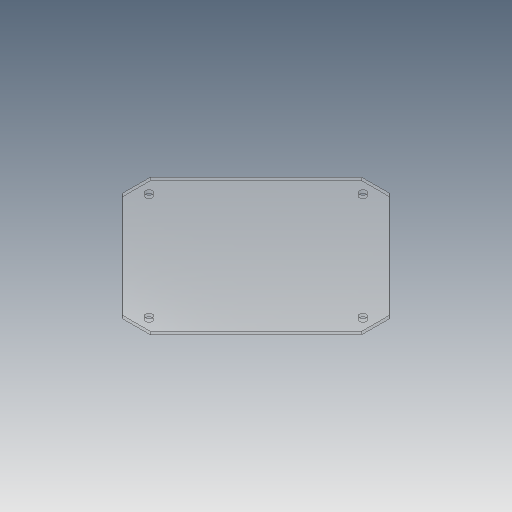
# Autodesk Inventor part: separatingPanels
Saved by Autodesk Inventor 2017 (Build 210142000, 142)
## iProperties
Created: 2016-07-21
Part Number: separatingPanels
Material: Polycarbonate, Clear
Document SubType Name: Modeling
Designer: Jonathan
Density: 1.2 g/cm^3
Appearance: Polycarbonate - Clear
Author: Jonathan
Autodesk Inventor part; units mm, degrees
ref_plane "YZ Plane" through (0, 0, 0) normal (1, 0, 0) x (0, 1, 0)
ref_plane "XZ Plane" through (0, 0, 0) normal (0, 1, 0) x (-1, 0, 0)
ref_plane "XY Plane" through (0, 0, 0) normal (0, 0, 1) x (1, 0, 0)
sketch "Sketch1" plane through (0, 0, 0) normal (0, 1, 0) x (-1, 0, 0)
  line L0 (95, -95) -> (-95, -95)
  line L1 (-95, -95) -> (-95, 95)
  line L2 (-95, 95) -> (95, 95)
  line L3 (95, 95) -> (95, -95)
  line L4 (95, -95) -> (-95, 95) construction
  line L5 (-95, -95) -> (95, 95) construction
  point P0 (0, 0)
  point P1 (0, 0)
  point P2 (0, 0)
  dimension "d25" = 190
  constraints: 12 end point, 3 midpoint, 2 parallel, 2 perpendicular, 1 coincident, 1 horizontal
  measures "d25" distance of L0.end L1.end
extrude "Extrusion1" add sketch "Sketch1" along normal blind 2.3813
sketch "Sketch2" plane through (0, 2.3813, 0) normal (0, 1, 0) x (1, 0, 0)
  line L0 (-95, -95) -> (95, -95) projected
  point P0 (0, 0)
  point P1 (0, -85)
  dimension "d26" = 10
  constraints: 1 vertical alignment
  measures "d26" distance from line of L0 point (0, -85)
hole "Hole1" at (0, 2.3813, 85) direction (0, -1, 0) diameter 5.5 end through all clearance for "Socket Head Cap Screw" size "M5" standard "Ansi Metric M Profile"
pattern_circular "Circular Pattern1" count 4 over 360 about axis through (0, -10, 0) along (0, 1, 0) of "Hole1"
sketch "Sketch3" plane through (0, 0, 0) normal (0, -1, 0) x (1, 0, 0)
  circle A0 centre (-85, 0) radius 2.75 projected
  circle A1 centre (0, -85) radius 2.75 projected
  circle A2 centre (85, 0) radius 2.75 projected
  circle A3 centre (0, 85) radius 2.75 projected
  line L0 (-95, -95) -> (95, -95) projected
  line L1 (95, -95) -> (95, 95) projected
  line L2 (95, 95) -> (-95, 95) projected
  line L3 (-95, 95) -> (-95, -95) projected
  line L4 (0, 106.066) -> (106.066, 0)
  line L5 (106.066, 0) -> (0, -106.066)
  line L6 (0, -106.066) -> (-106.066, 0)
  line L7 (-106.066, 0) -> (0, 106.066)
  line L8 (-106.066, 0) -> (106.066, 0) construction
  line L9 (0, -106.066) -> (0, 106.066) construction
  point P0 (0, 0)
  point P1 (0, 0)
  point P2 (0, 0)
  dimension "d27" = 150
  dimension "d28" = 150
  constraints: 12 end point, 2 midpoint, 2 parallel, 1 coincident, 1 horizontal, 1 perpendicular
  measures "d27" distance between parallel lines of L7 L5
  measures "d28" distance between parallel lines of L6 L4
extrude "Extrusion2" cut sketch "Sketch3" against normal through all contours L6 L3 L7 L2 L4 L1 L5 L0 | L0 L5 L6 | L6 L7 L3 | L1 L4 L5 | L7 L4 L2 keep common part
equation "\"d7\" = suppourtPanelThickness"
equation "\"d28\" = d27"
equation "\"panelChamfer\" = 75"
equation "\"suppourtPanelThickness\" = 2.38125"
body "Solid1"
